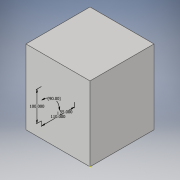
# Autodesk Inventor part: Tower
Saved by Autodesk Inventor 2018 (Build 220112000, 112)
## iProperties
Created: 2019-01-28
Part Number: Tower
Material: Generic
Document SubType Name: Modeling
Designer: This kid
Density: 1 g/cm^3
Appearance: Default
Author: This kid
Autodesk Inventor part; units mm, degrees
ref_plane "YZ Plane" through (0, 0, 0) normal (1, 0, 0) x (0, 1, 0)
ref_plane "XZ Plane" through (0, 0, 0) normal (0, 1, 0) x (-1, 0, 0)
ref_plane "XY Plane" through (0, 0, 0) normal (0, 0, 1) x (1, 0, 0)
sketch "Sketch1" plane through (0, 0, 0) normal (0, 1, 0) x (-1, 0, 0)
  point P0 (0, 0)
sketch "Sketch2" plane through (0, 0, 0) normal (0, 1, 0) x (-1, 0, 0)
  line L0 (0, 0) -> (5471.6222, 0)
  line L1 (5471.6222, 0) -> (5471.6222, -5471.6222)
  line L2 (5471.6222, -5471.6222) -> (0, -5471.6222)
  line L3 (0, -5471.6222) -> (0, 0)
  dimension "d0" = 5471.6222
  dimension "d1" = 5471.6222
  constraints: 8 end point, 2 parallel, 1 horizontal, 1 perpendicular
  measures "d0" distance of L1.end L2.end
  measures "d1" distance of L0.end L1.end
extrude "Extrusion1" add sketch "Sketch2" along normal blind 6350
sketch "Sketch3" plane through (-5471.6222, 0, -5471.6222) normal (-1, 0, 0) x (0, 0, 1)
  line L0 (0, 0) -> (5471.6222, 0) projected
  line L1 (2735.8111, 0) -> (1338.8111, 0)
  line L2 (1338.8111, 0) -> (4132.8111, 0)
  line L3 (4132.8111, 0) -> (4132.8111, 2540)
  line L4 (4132.8111, 2540) -> (1338.8111, 2540)
  line L5 (1338.8111, 2540) -> (1338.8111, 0)
  dimension "d4" = 1397
  dimension "d5" = 2794
  dimension "d6" = 2540
  dimension "d7" = 90
  constraints: 10 end point, 3 perpendicular, 2 point on line, 1 midpoint
  measures "d4" distance of L1.start L1.end
  measures "d5" distance of L1.end L2.end
  measures "d6" distance of L2.end L3.end
  measures "d7" angle of L3 L2
body "Solid1"
